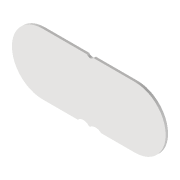
# Autodesk Inventor part: Bauteil2
Saved by Autodesk Inventor 2021 (Build 250183000, 183)
## iProperties
Created: 2021-09-11
Part Number: Bauteil2
Material: Generisch
Document SubType Name: Modeling
Designer: Rama
Density: 1 g/cm^3
Appearance: Vorgabe
Author: Rama
Autodesk Inventor part; units mm, degrees
ref_plane "YZ Plane" through (0, 0, 0) normal (1, 0, 0) x (0, 1, 0)
ref_plane "XZ Plane" through (0, 0, 0) normal (0, 1, 0) x (-1, 0, 0)
sketch "Skizze1" plane through (0, 0, 0) normal (0, 0, 1) x (1, 0, 0)
  circle A0 centre (32, 0) radius 22.5
  circle A1 centre (-36, 0) radius 22.5
  line L0 (-36, -22.5) -> (32, -22.5)
  line L1 (-36, 22.5) -> (32, 22.5)
  circle A2 centre (-6, -26) radius 5.3852
  circle A3 centre (3, -27) radius 6.0828
  circle A4 centre (-1, 24) radius 2.8875
  point P0 (0, 0)
  point P1 (-10.0927, -22.5)
  point P2 (-1.9073, -22.5)
  point P3 (-1.0927, -22.5)
  point P4 (7.0927, -22.5)
  point P5 (1.4674, 22.5)
  point P6 (-3.4674, 22.5)
  dimension "d1" = 45
  dimension "d2" = 45
  dimension "d3" = 68
  dimension "d4" = 0
  constraints: 5 centre point, 4 end point, 4 point on circle, 4 tangent
  measures "d1" diameter of A0
  measures "d2" diameter of A1
  measures "d3" distance of A1.centre A0.centre
  measures "d4" vertical distance of A1.centre A0.centre
ref_plane "Arbeitsebene1" through (-62.5751, -29.26, -1.7438) normal (0, 0, -1) x (0, 1, 0)
extrude "Extrusion1" add sketch "Skizze1" against normal up to surface (1.7438 mm away) contours A0 | A0 L0 A3 A2 A1 L1 A4 | A1
equation "\"d2\" = d1"
